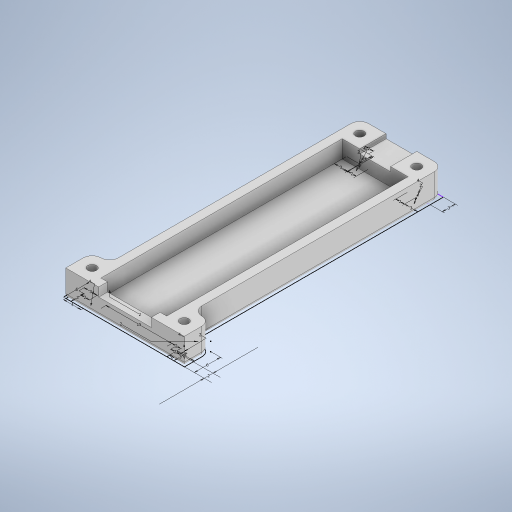
# Autodesk Inventor part: Case Atas
Saved by Autodesk Inventor 2024 (Build 280153000, 153)
## iProperties
Created: 2023-08-08
Part Number: Case Atas
Material: Generic
Document SubType Name: Modeling
Designer: Asus
Density: 1 g/cm^3
Appearance: Default
Author: Asus
## iProperties of the stored document Case Atas_3DPrint.ipt
Created: 2023-08-08
Part Number: Case Atas_3DPrint
Material: Generic
Document SubType Name: Modeling
Designer: Asus
Density: 1 g/cm^3
Appearance: Default
Author: Asus
Autodesk Inventor part; units mm, degrees
(part 1 of 2)
ref_plane "YZ Plane" through (0, 0, 0) normal (1, 0, 0) x (0, 1, 0)
ref_plane "XZ Plane" through (0, 0, 0) normal (0, 1, 0) x (-1, 0, 0)
ref_plane "XY Plane" through (0, 0, 0) normal (0, 0, 1) x (1, 0, 0)
sketch "Sketch2" plane through (0, 0, 0) normal (0, 1, 0) x (-1, 0, 0)
  line L0 (0, 0) -> (0, -2)
  line L1 (0, -2) -> (2, -2) construction
  line L2 (2, -2) -> (17, -2) construction
  line L3 (17, -2) -> (17, -57) construction
  line L4 (2, -2) -> (17, -2)
  line L5 (17, -2) -> (17, -57)
  line L6 (17, -57) -> (2, -57)
  line L7 (2, -57) -> (2, -2)
  line L8 (17, -57) -> (17, -63) construction
  line L9 (17, -63) -> (19, -63) construction
  line L10 (0, 0) -> (19, 0)
  line L11 (19, -8) -> (19, -63)
  line L12 (19, -63) -> (0, -63)
  line L13 (0, -63) -> (0, -8)
  line L14 (19, 0) -> (23, 0)
  line L15 (23, 0) -> (23, -4)
  line L16 (21, -6) -> (21, -6)
  arc A0 (21, -6) -> (19, -8) centre (21, -8) ccw
  arc A1 (21, -6) -> (23, -4) centre (21, -4) ccw
  line L17 (0, 0) -> (-4, 0)
  line L18 (-4, 0) -> (-4, -4)
  line L19 (-2, -6) -> (-2, -6)
  arc A2 (0, -8) -> (-2, -6) centre (-2, -8) ccw
  arc A3 (-4, -4) -> (-2, -6) centre (-2, -4) ccw
  line L20 (23, 0) -> (23, -3) construction
  line L21 (0, 0) -> (-1, 0) construction
  line L22 (-1, 0) -> (-1, -3) construction
  circle A4 centre (-1, -3) radius 1
  line L23 (23, 0) -> (23, -3) construction
  line L24 (23, -3) -> (20, -3) construction
  line L25 (20, -3) -> (22, -3) construction
  circle A5 centre (20, -3) radius 1
  line L26 (-1, -3) -> (1, -3) construction
  line L27 (0, -63) -> (0, -60) construction
  line L28 (0, -60) -> (3, -60) construction
  line L29 (19, -63) -> (19, -60) construction
  line L30 (19, -60) -> (16, -60) construction
  line L31 (16, -60) -> (14, -60) construction
  line L32 (3, -60) -> (5, -60) construction
  circle A6 centre (3, -60) radius 1
  circle A7 centre (16, -60) radius 1
  circle A8 centre (-1, -3) radius 2
  circle A9 centre (20, -3) radius 2
  circle A10 centre (3, -60) radius 2
  circle A11 centre (16, -60) radius 2
  point P0 (23, -6)
  point P1 (-4, -6)
  dimension "d4" = 2
  dimension "d5" = 2
  dimension "d6" = 15
  dimension "d8" = 6
  dimension "d9" = 2
  dimension "d15" = 4
  dimension "d16" = 6
  dimension "d17" = 2
  dimension "d18" = 4
  dimension "d19" = 6
  dimension "d20" = 2
  dimension "d34" = 1
  dimension "d35" = 3
  dimension "d36" = 2
  dimension "d39" = 3
  dimension "d40" = 3
  dimension "d41" = 2
  dimension "d43" = 2
  dimension "d52" = 3
  dimension "d53" = 3
  dimension "d54" = 3
  dimension "d55" = 3
  dimension "d56" = 2
  dimension "d57" = 2
  dimension "d58" = 2
  dimension "d59" = 2
  dimension "d73" = 4
  dimension "d74" = 4
  dimension "d75" = 4
  dimension "d76" = 4
  constraints: 66 end point, 15 point on line, 13 perpendicular, 12 centre point, 12 coincident, 8 point on circle, 8 tangent, 5 horizontal, 4 parallel, 2 equal radius, 2 vertical
  measures "d4" distance of L0.start L0.end
  measures "d5" distance of L0.end L1.end
  measures "d6" distance of L1.end L2.end
  measures "d8" distance of L3.end L8.end
  measures "d9" distance of L8.end L9.end
  measures "d15" distance of L10.end L14.end
  measures "d16" distance of L14.end point (23, -6)
  measures "d17" radius of A0
  measures "d18" distance of L0.start L17.end
  measures "d19" distance of L17.end point (-4, -6)
  measures "d20" radius of A2
  measures "d34" distance of L0.start L21.end
  measures "d35" distance of L21.end L22.end
  measures "d36" diameter of A4
  measures "d39" distance of L14.end L20.end
  measures "d40" distance of L20.end L24.end
  measures "d41" distance of L24.end L25.end
  measures "d43" distance of L26.start L26.end
  measures "d52" distance of L12.end L27.end
  measures "d53" distance of L27.end L28.end
  measures "d54" distance of L9.end L29.end
  measures "d55" distance of L29.end L30.end
  measures "d56" distance of L30.end L31.end
  measures "d57" distance of L28.end L32.end
  measures "d58" diameter of A6
  measures "d59" diameter of A7
  measures "d73" diameter of A8
  measures "d74" diameter of A9
  measures "d75" diameter of A10
  measures "d76" diameter of A11
extrude "Extrusion7" add sketch "Sketch2" along normal blind 6 contours L10 L14 L15 A1 A0 L11 L12 L13 A2 A3 L18 L17 | A4 | A5 | A8 | A9 | A10 | A11
extrude "Extrusion9" add sketch "Sketch2" along normal blind 2 contours L4 L5 L6 L7
sketch "Sketch7" plane through (-23, 0, 0) normal (0, 0, 1) x (1, 0, 0)
  line L0 (0, 0) -> (0, 6) construction
  line L1 (0, 6) -> (27, 6) construction
  line L2 (0, 6) -> (27, 6) construction
  line L3 (13.5, 6) -> (13.5, 4) construction
  line L4 (13.5, 4) -> (19.5, 4) construction
  line L5 (19.5, 4) -> (7.5, 4)
  line L6 (7.5, 4) -> (7.5, 6)
  line L7 (7.5, 6) -> (19.5, 6)
  line L8 (19.5, 6) -> (19.5, 4)
  point P0 (23, 0)
  dimension "d62" = 2
  dimension "d63" = 6
  dimension "d64" = 12
  constraints: 14 end point, 3 parallel, 1 collinear, 1 horizontal, 1 midpoint, 1 perpendicular, 1 point on line, 1 vertical
  measures "d62" distance of L3.start L3.end
  measures "d63" distance of L3.end L4.end
  measures "d64" distance of L6.end L7.end
extrude "Extrusion10" cut sketch "Sketch7" against normal blind 2
sketch "Sketch9" plane through (0, 0, -63) normal (0, 0, -1) x (-1, 0, 0)
  line L0 (0, 0) -> (0, 6) construction
  line L1 (0, 6) -> (19, 6) construction
  line L2 (0, 6) -> (19, 6) construction
  line L3 (9.5, 6) -> (9.5, 5) construction
  line L4 (9.5, 5) -> (13, 5) construction
  line L5 (13, 5) -> (6, 5)
  line L6 (6, 5) -> (6, 6)
  line L7 (6, 6) -> (13, 6)
  line L8 (13, 6) -> (13, 5)
  dimension "d67" = 1
  dimension "d68" = 3.5
  dimension "d69" = 7
  constraints: 14 end point, 3 equal length, 2 perpendicular, 1 horizontal, 1 midpoint, 1 point on line, 1 vertical
  measures "d67" distance of L3.start L3.end
  measures "d68" distance of L3.end L4.end
  measures "d69" distance of L6.end L7.end
extrude "Extrusion11" cut sketch "Sketch9" against normal blind 6
fillet "Fillet1" radius 2 2 edges at (0, 3, -63) (-19, 3, -63)
extrude "Extrusion12" cut sketch "Sketch2" along normal blind 1 contours A4 | A5 | A6 | A7 | A8 | A9 | A10 | A11
extrude "Extrusion13" cut sketch "Sketch2" along normal blind 6 contours A4 | A5
fillet "Fillet2" radius 0.9 12 edges at (-0.5858, 0, -62.4142) (-9.5, 0, -63) (-18.4142, 0, -62.4142) (-19, 0, -34.5) (-19.5858, 0, -6.5858) (-22.4142, 0, -5.4142) (-23, 0, -2) (0.5858, 0, -6.5858) (3.4142, 0, -5.4142) (4, 0, -2) (0, 0, -34.5) (-9.5, 0, 0)
sketch "Sketch10" plane through (0, 0, 0) normal (0, -1, 0) x (1, 0, 0)
  line L0 (-5.0264, -9.1176) -> (-5.0264, -52.1576) construction
  line L1 (-5.0264, -52.1576) -> (-18.2298, -52.1576) construction
  line L2 (-18.2298, -52.1576) -> (-18.2298, -9.1176) construction
  line L3 (-18.2298, -9.1176) -> (-5.0264, -9.1176) construction
  line L4 (-5.0599, -17.9524) -> (-5.0599, -18.3563)
  line L5 (-5.0599, -18.3563) -> (-6.1437, -18.3563)
  spline S0 degree 2 poles (-6.1437, -18.3563) (-6.4014, -18.3563) (-6.4776, -18.3716) knots 0 0 0 1 1 1
  spline S1 degree 2 poles (-6.4776, -18.3716) (-6.5995, -18.3975) (-6.7489, -18.5926) (-6.7489, -18.7618) knots 0 0 0 1 2 2 2
  spline S2 degree 2 poles (-6.7489, -18.7618) (-6.7489, -18.9326) (-6.6087, -19.1079) (-6.4044, -19.1429) (-6.1666, -19.1429) knots 0 0 0 1 2 3 3 3
  line L6 (-6.1666, -19.1429) -> (-5.0599, -19.1429)
  line L7 (-5.0599, -19.1429) -> (-5.0599, -19.5469)
  line L8 (-5.0599, -19.5469) -> (-6.1102, -19.5469)
  spline S3 degree 2 poles (-6.1102, -19.5469) (-6.47, -19.5469) (-6.7672, -19.4813) (-6.9715, -19.306) (-7.0934, -19.0103) (-7.0934, -18.774) knots 0 0 0 1 2 3 4 4 4
  spline S4 degree 2 poles (-7.0934, -18.774) (-7.0934, -18.4874) (-6.9608, -18.1917) (-6.7504, -18.0194) (-6.6331, -17.992) knots 0 0 0 1 2 3 3 3
  spline S5 degree 2 poles (-6.6331, -17.992) (-6.4623, -17.9524) (-6.127, -17.9524) knots 0 0 0 1 1 1
  line L9 (-6.127, -17.9524) -> (-5.0599, -17.9524)
  line L10 (-6.4075, -19.8701) -> (-6.3693, -20.2633)
  spline S6 degree 2 poles (-6.3693, -20.2633) (-6.5675, -20.2984) (-6.7535, -20.5164) (-6.7535, -20.6993) knots 0 0 0 1 2 2 2
  spline S7 degree 2 poles (-6.7535, -20.6993) (-6.7535, -20.8944) (-6.5889, -21.0926) (-6.4776, -21.0926) knots 0 0 0 1 2 2 2
  spline S8 degree 2 poles (-6.4776, -21.0926) (-6.4059, -21.0926) (-6.3068, -21.0088) (-6.2703, -20.9051) knots 0 0 0 1 2 2 2
  spline S9 degree 2 poles (-6.2703, -20.9051) (-6.2459, -20.835) (-6.1834, -20.5819) knots 0 0 0 1 1 1
  spline S10 degree 2 poles (-6.1834, -20.5819) (-6.1026, -20.2572) (-5.9852, -20.1262) knots 0 0 0 1 1 1
  spline S11 degree 2 poles (-5.9852, -20.1262) (-5.8206, -19.9417) (-5.5843, -19.9417) knots 0 0 0 1 1 1
  spline S12 degree 2 poles (-5.5843, -19.9417) (-5.4303, -19.9417) (-5.1651, -20.1155) (-5.0264, -20.4417) (-5.0264, -20.6719) knots 0 0 0 1 2 3 3 3
  spline S13 degree 2 poles (-5.0264, -20.6719) (-5.0264, -21.0484) (-5.3556, -21.4295) (-5.6315, -21.4387) knots 0 0 0 1 2 2 2
  line L11 (-5.6315, -21.4387) -> (-5.6498, -21.0347)
  spline S14 degree 2 poles (-5.6498, -21.0347) (-5.4959, -21.0088) (-5.3602, -20.838) (-5.3602, -20.6673) knots 0 0 0 1 2 2 2
  spline S15 degree 2 poles (-5.3602, -20.6673) (-5.3602, -20.4905) (-5.4318, -20.3914) knots 0 0 0 1 1 1
  spline S16 degree 2 poles (-5.4318, -20.3914) (-5.4791, -20.3274) (-5.5568, -20.3274) knots 0 0 0 1 1 1
  spline S17 degree 2 poles (-5.5568, -20.3274) (-5.627, -20.3274) (-5.6788, -20.3868) knots 0 0 0 1 1 1
  spline S18 degree 2 poles (-5.6788, -20.3868) (-5.7428, -20.4646) (-5.8815, -21.0545) (-6.0294, -21.3365) (-6.287, -21.4966) (-6.4776, -21.4966) knots 0 0 0 1 2 3 4 4 4
  spline S19 degree 2 poles (-6.4776, -21.4966) (-6.6483, -21.4966) (-6.9486, -21.306) (-7.095, -20.9569) (-7.095, -20.6963) knots 0 0 0 1 2 3 3 3
  spline S20 degree 2 poles (-7.095, -20.6963) (-7.095, -20.3167) (-6.7443, -19.9097) (-6.4075, -19.8701) knots 0 0 0 1 2 2 2
  line L12 (-5.0599, -21.838) -> (-5.0599, -22.6383)
  spline S21 degree 2 poles (-5.0599, -22.6383) (-5.0599, -22.8762) (-5.0995, -23.1094) (-5.2245, -23.2938) (-5.4334, -23.4173) (-5.5629, -23.4173) knots 0 0 0 1 2 3 4 4 4
  spline S22 degree 2 poles (-5.5629, -23.4173) (-5.7032, -23.4173) (-5.9364, -23.2664) (-5.9959, -23.1368) knots 0 0 0 1 2 2 2
  spline S23 degree 2 poles (-5.9959, -23.1368) (-6.0492, -23.3197) (-6.3053, -23.5149) (-6.4791, -23.5149) knots 0 0 0 1 2 2 2
  spline S24 degree 2 poles (-6.4791, -23.5149) (-6.6163, -23.5149) (-6.8739, -23.3883) (-7.0279, -23.1673) (-7.0462, -23.0072) knots 0 0 0 1 2 3 3 3
  spline S25 degree 2 poles (-7.0462, -23.0072) (-7.0568, -22.9051) (-7.0599, -22.5194) knots 0 0 0 1 1 1
  line L13 (-7.0599, -22.5194) -> (-7.0599, -21.838)
  line L14 (-7.0599, -21.838) -> (-5.0599, -21.838)
  line L15 (-6.1864, -22.242) -> (-6.7215, -22.242)
  line L16 (-6.7215, -22.242) -> (-6.7215, -22.617)
  spline S26 degree 2 poles (-6.7215, -22.617) (-6.7215, -22.8365) (-6.7093, -22.8944) knots 0 0 0 1 1 1
  spline S27 degree 2 poles (-6.7093, -22.8944) (-6.6925, -22.9844) (-6.566, -23.0987) (-6.4593, -23.0987) knots 0 0 0 1 2 2 2
  spline S28 degree 2 poles (-6.4593, -23.0987) (-6.3693, -23.0987) (-6.2443, -23.0118) (-6.1864, -22.8457) (-6.1864, -22.5697) knots 0 0 0 1 2 3 3 3
  line L17 (-6.1864, -22.5697) -> (-6.1864, -22.242)
  line L18 (-5.3922, -22.242) -> (-5.8541, -22.242)
  line L19 (-5.8541, -22.242) -> (-5.8541, -22.5072)
  spline S29 degree 2 poles (-5.8541, -22.5072) (-5.8541, -22.7435) (-5.848, -22.8015) knots 0 0 0 1 1 1
  spline S30 degree 2 poles (-5.848, -22.8015) (-5.8343, -22.9051) (-5.7169, -23.024) (-5.6193, -23.024) knots 0 0 0 1 2 2 2
  spline S31 degree 2 poles (-5.6193, -23.024) (-5.5264, -23.024) (-5.412, -22.9219) (-5.3983, -22.8197) knots 0 0 0 1 2 2 2
  spline S32 degree 2 poles (-5.3983, -22.8197) (-5.3922, -22.7603) (-5.3922, -22.4737) knots 0 0 0 1 1 1
  line L20 (-5.3922, -22.4737) -> (-5.3922, -22.242)
  line L21 (-5.6102, -25.2923) -> (-5.9151, -25.2923)
  line L22 (-5.9151, -25.2923) -> (-5.9151, -25.0301)
  line L23 (-5.9151, -25.0301) -> (-6.4989, -25.0301)
  spline S33 degree 2 poles (-6.4989, -25.0301) (-6.6757, -25.0301) (-6.7352, -25.0454) (-6.7733, -25.0987) (-6.7733, -25.1368) knots 0 0 0 1 2 3 3 3
  spline S34 degree 2 poles (-6.7733, -25.1368) (-6.7733, -25.1902) (-6.7367, -25.2923) knots 0 0 0 1 1 1
  line L24 (-6.7367, -25.2923) -> (-7.034, -25.3243)
  spline S35 degree 2 poles (-7.034, -25.3243) (-7.0919, -25.1902) (-7.0919, -25.021) knots 0 0 0 1 1 1
  spline S36 degree 2 poles (-7.0919, -25.021) (-7.0919, -24.9173) (-7.0218, -24.7512) (-6.912, -24.6734) (-6.8175, -24.6582) knots 0 0 0 1 2 3 3 3
  spline S37 degree 2 poles (-6.8175, -24.6582) (-6.7504, -24.646) (-6.5477, -24.646) knots 0 0 0 1 1 1
  line L25 (-6.5477, -24.646) -> (-5.9151, -24.646)
  line L26 (-5.9151, -24.646) -> (-5.9151, -24.4707)
  line L27 (-5.9151, -24.4707) -> (-5.6102, -24.4707)
  line L28 (-5.6102, -24.4707) -> (-5.6102, -24.646)
  line L29 (-5.6102, -24.646) -> (-5.3221, -24.646)
  line L30 (-5.3221, -24.646) -> (-5.0965, -25.0301)
  line L31 (-5.0965, -25.0301) -> (-5.6102, -25.0301)
  line L32 (-5.6102, -25.0301) -> (-5.6102, -25.2923)
  spline S38 degree 2 poles (-6.3145, -25.4691) (-6.1239, -25.4691) (-5.7657, -25.6582) (-5.5782, -26.0027) (-5.5782, -26.2161) knots 0 0 0 1 2 3 3 3
  spline S39 degree 2 poles (-5.5782, -26.2161) (-5.5782, -26.5454) (-6.005, -26.9661) (-6.3312, -26.9661) knots 0 0 0 1 2 2 2
  spline S40 degree 2 poles (-6.3312, -26.9661) (-6.659, -26.9661) (-7.0919, -26.5408) (-7.0919, -26.2191) knots 0 0 0 1 2 2 2
  spline S41 degree 2 poles (-7.0919, -26.2191) (-7.0919, -26.0194) (-6.912, -25.6582) (-6.5645, -25.4691) (-6.3145, -25.4691) knots 0 0 0 1 2 3 3 3
  spline S42 degree 2 poles (-6.3343, -25.8624) (-6.5507, -25.8624) (-6.7794, -26.0667) (-6.7794, -26.2176) knots 0 0 0 1 2 2 2
  spline S43 degree 2 poles (-6.7794, -26.2176) (-6.7794, -26.3685) (-6.5507, -26.5713) (-6.3328, -26.5713) knots 0 0 0 1 2 2 2
  spline S44 degree 2 poles (-6.3328, -26.5713) (-6.1193, -26.5713) (-5.8907, -26.3685) (-5.8907, -26.2176) knots 0 0 0 1 2 2 2
  spline S45 degree 2 poles (-5.8907, -26.2176) (-5.8907, -26.0667) (-6.1193, -25.8624) (-6.3343, -25.8624) knots 0 0 0 1 2 2 2
  line L33 (-7.0599, -28.4951) -> (-5.3983, -28.4951)
  line L34 (-5.3983, -28.4951) -> (-5.3983, -27.9021)
  line L35 (-5.3983, -27.9021) -> (-5.0599, -27.9021)
  line L36 (-5.0599, -27.9021) -> (-5.0599, -29.4905)
  line L37 (-5.0599, -29.4905) -> (-5.3983, -29.4905)
  line L38 (-5.3983, -29.4905) -> (-5.3983, -28.899)
  line L39 (-5.3983, -28.899) -> (-7.0599, -28.899)
  line L40 (-7.0599, -28.899) -> (-7.0599, -28.4951)
  line L41 (-7.0599, -30.2024) -> (-5.3983, -30.2024)
  line L42 (-5.3983, -30.2024) -> (-5.3983, -29.6094)
  line L43 (-5.3983, -29.6094) -> (-5.0599, -29.6094)
  line L44 (-5.0599, -29.6094) -> (-5.0599, -31.1978)
  line L45 (-5.0599, -31.1978) -> (-5.3983, -31.1978)
  line L46 (-5.3983, -31.1978) -> (-5.3983, -30.6063)
  line L47 (-5.3983, -30.6063) -> (-7.0599, -30.6063)
  line L48 (-7.0599, -30.6063) -> (-7.0599, -30.2024)
  line L49 (-7.0599, -31.4707) -> (-5.0767, -31.4707)
  line L50 (-5.0767, -31.4707) -> (-5.0767, -31.8746)
  line L51 (-5.0767, -31.8746) -> (-6.7215, -31.8746)
  line L52 (-6.7215, -31.8746) -> (-6.7215, -32.8792)
  line L53 (-6.7215, -32.8792) -> (-7.0599, -32.8792)
  line L54 (-7.0599, -32.8792) -> (-7.0599, -31.4707)
  line L55 (-7.0599, -33.9432) -> (-5.0599, -33.9432)
  line L56 (-5.0599, -33.9432) -> (-5.0599, -34.5911)
  spline S46 degree 2 poles (-5.0599, -34.5911) (-5.0599, -34.96) (-5.0904, -35.0713) knots 0 0 0 1 1 1
  spline S47 degree 2 poles (-5.0904, -35.0713) (-5.1346, -35.2435) (-5.4364, -35.4752) (-5.6757, -35.4752) knots 0 0 0 1 2 2 2
  spline S48 degree 2 poles (-5.6757, -35.4752) (-5.8587, -35.4752) (-6.1102, -35.3411) (-6.2535, -35.1353) (-6.2764, -35.0286) knots 0 0 0 1 2 3 3 3
  spline S49 degree 2 poles (-6.2764, -35.0286) (-6.3053, -34.8853) (-6.3053, -34.6109) knots 0 0 0 1 1 1
  line L57 (-6.3053, -34.6109) -> (-6.3053, -34.3472)
  line L58 (-6.3053, -34.3472) -> (-7.0599, -34.3472)
  line L59 (-7.0599, -34.3472) -> (-7.0599, -33.9432)
  line L60 (-5.3983, -34.3472) -> (-5.9669, -34.3472)
  line L61 (-5.9669, -34.3472) -> (-5.9669, -34.5682)
  spline S50 degree 2 poles (-5.9669, -34.5682) (-5.9669, -34.8076) (-5.9044, -34.9676) (-5.7703, -35.0591) (-5.6818, -35.0591) knots 0 0 0 1 2 3 3 3
  spline S51 degree 2 poles (-5.6818, -35.0591) (-5.5721, -35.0591) (-5.4303, -34.931) (-5.412, -34.8319) knots 0 0 0 1 2 2 2
  spline S52 degree 2 poles (-5.412, -34.8319) (-5.3983, -34.7603) (-5.3983, -34.5423) knots 0 0 0 1 1 1
  line L62 (-5.3983, -34.5423) -> (-5.3983, -34.3472)
  line L63 (-7.0599, -35.8182) -> (-5.0767, -35.8182)
  line L64 (-5.0767, -35.8182) -> (-5.0767, -36.2222)
  line L65 (-5.0767, -36.2222) -> (-6.7215, -36.2222)
  line L66 (-6.7215, -36.2222) -> (-6.7215, -37.2268)
  line L67 (-6.7215, -37.2268) -> (-7.0599, -37.2268)
  line L68 (-7.0599, -37.2268) -> (-7.0599, -35.8182)
  line L69 (-6.7032, -38.7237) -> (-7.0599, -38.7237)
  line L70 (-7.0599, -38.7237) -> (-7.0599, -37.3807)
  spline S53 degree 2 poles (-7.0599, -37.3807) (-6.8587, -37.4021) (-6.4974, -37.6201) (-6.1986, -37.9432) knots 0 0 0 1 2 2 2
  spline S54 degree 2 poles (-6.1986, -37.9432) (-5.9578, -38.2024) (-5.8709, -38.2603) knots 0 0 0 1 1 1
  spline S55 degree 2 poles (-5.8709, -38.2603) (-5.752, -38.3396) (-5.6361, -38.3396) knots 0 0 0 1 1 1
  spline S56 degree 2 poles (-5.6361, -38.3396) (-5.5081, -38.3396) (-5.3709, -38.2024) (-5.3709, -38.0804) knots 0 0 0 1 2 2 2
  spline S57 degree 2 poles (-5.3709, -38.0804) (-5.3709, -37.9615) (-5.5157, -37.8197) (-5.6834, -37.8091) knots 0 0 0 1 2 2 2
  line L71 (-5.6834, -37.8091) -> (-5.6453, -37.4265)
  spline S58 degree 2 poles (-5.6453, -37.4265) (-5.3282, -37.46) (-5.0523, -37.8197) (-5.0523, -38.0896) knots 0 0 0 1 2 2 2
  spline S59 degree 2 poles (-5.0523, -38.0896) (-5.0523, -38.3853) (-5.3709, -38.7237) (-5.6087, -38.7237) knots 0 0 0 1 2 2 2
  spline S60 degree 2 poles (-5.6087, -38.7237) (-5.7428, -38.7237) (-5.9867, -38.6277) (-6.1209, -38.5225) knots 0 0 0 1 2 2 2
  spline S61 degree 2 poles (-6.1209, -38.5225) (-6.2093, -38.4524) (-6.5416, -38.0896) (-6.6514, -37.992) (-6.7032, -37.963) knots 0 0 0 1 2 3 3 3
  line L72 (-6.7032, -37.963) -> (-6.7032, -38.7237)
  line L73 (-6.5279, -38.9691) -> (-6.4821, -39.3396)
  spline S62 degree 2 poles (-6.4821, -39.3396) (-6.6239, -39.3579) (-6.7748, -39.5133) (-6.7748, -39.6231) knots 0 0 0 1 2 2 2
  spline S63 degree 2 poles (-6.7748, -39.6231) (-6.7748, -39.742) (-6.595, -39.9036) (-6.4425, -39.9036) knots 0 0 0 1 2 2 2
  spline S64 degree 2 poles (-6.4425, -39.9036) (-6.2977, -39.9036) (-6.1285, -39.7496) (-6.1285, -39.6383) knots 0 0 0 1 2 2 2
  spline S65 degree 2 poles (-6.1285, -39.6383) (-6.1285, -39.5652) (-6.1575, -39.463) knots 0 0 0 1 1 1
  line L74 (-6.1575, -39.463) -> (-5.845, -39.5057)
  spline S66 degree 2 poles (-5.845, -39.5057) (-5.8495, -39.6612) (-5.7062, -39.8243) (-5.5873, -39.8243) knots 0 0 0 1 2 2 2
  spline S67 degree 2 poles (-5.5873, -39.8243) (-5.4867, -39.8243) (-5.3678, -39.7039) (-5.3678, -39.6048) knots 0 0 0 1 2 2 2
  spline S68 degree 2 poles (-5.3678, -39.6048) (-5.3678, -39.5057) (-5.5035, -39.367) (-5.6346, -39.3518) knots 0 0 0 1 2 2 2
  line L75 (-5.6346, -39.3518) -> (-5.5751, -38.9981)
  spline S69 degree 2 poles (-5.5751, -38.9981) (-5.3937, -39.0347) (-5.1757, -39.1841) (-5.0523, -39.4493) (-5.0523, -39.6155) knots 0 0 0 1 2 3 3 3
  spline S70 degree 2 poles (-5.0523, -39.6155) (-5.0523, -39.8975) (-5.2321, -40.0682) knots 0 0 0 1 1 1
  spline S71 degree 2 poles (-5.2321, -40.0682) (-5.3785, -40.2085) (-5.5645, -40.2085) knots 0 0 0 1 1 1
  spline S72 degree 2 poles (-5.5645, -40.2085) (-5.8267, -40.2085) (-5.9837, -39.9204) knots 0 0 0 1 1 1
  spline S73 degree 2 poles (-5.9837, -39.9204) (-6.0203, -40.0926) (-6.2779, -40.2969) (-6.4593, -40.2969) knots 0 0 0 1 2 2 2
  spline S74 degree 2 poles (-6.4593, -40.2969) (-6.723, -40.2969) (-7.0934, -39.9127) (-7.0934, -39.6262) knots 0 0 0 1 2 2 2
  spline S75 degree 2 poles (-7.0934, -39.6262) (-7.0934, -39.3548) (-6.7809, -38.9981) (-6.5279, -38.9691) knots 0 0 0 1 2 2 2
  spline S76 degree 2 poles (-5.0523, -41.1841) (-5.0523, -41.4752) (-5.2596, -41.6383) knots 0 0 0 1 1 1
  spline S77 degree 2 poles (-5.2596, -41.6383) (-5.505, -41.8335) (-6.0736, -41.8335) knots 0 0 0 1 1 1
  spline S78 degree 2 poles (-6.0736, -41.8335) (-6.6407, -41.8335) (-6.8892, -41.6368) knots 0 0 0 1 1 1
  spline S79 degree 2 poles (-6.8892, -41.6368) (-7.0934, -41.4752) (-7.0934, -41.1841) knots 0 0 0 1 1 1
  spline S80 degree 2 poles (-7.0934, -41.1841) (-7.0934, -40.8914) (-6.6453, -40.5347) (-6.069, -40.5347) knots 0 0 0 1 2 2 2
  spline S81 degree 2 poles (-6.069, -40.5347) (-5.505, -40.5347) (-5.2565, -40.7313) knots 0 0 0 1 1 1
  spline S82 degree 2 poles (-5.2565, -40.7313) (-5.0523, -40.8929) (-5.0523, -41.1841) knots 0 0 0 1 1 1
  spline S83 degree 2 poles (-5.3709, -41.1841) (-5.3709, -41.114) (-5.4593, -41.0057) (-5.5736, -40.9752) knots 0 0 0 1 2 2 2
  spline S84 degree 2 poles (-5.5736, -40.9752) (-5.7215, -40.9356) (-6.0736, -40.9356) knots 0 0 0 1 1 1
  spline S85 degree 2 poles (-6.0736, -40.9356) (-6.4242, -40.9356) (-6.6879, -41.0072) (-6.7748, -41.114) (-6.7748, -41.1841) knots 0 0 0 1 2 3 3 3
  spline S86 degree 2 poles (-6.7748, -41.1841) (-6.7748, -41.2542) (-6.6864, -41.3624) (-6.5721, -41.3929) knots 0 0 0 1 2 2 2
  spline S87 degree 2 poles (-6.5721, -41.3929) (-6.4242, -41.4326) (-6.0736, -41.4326) knots 0 0 0 1 1 1
  spline S88 degree 2 poles (-6.0736, -41.4326) (-5.7215, -41.4326) (-5.4593, -41.3609) (-5.3709, -41.2542) (-5.3709, -41.1841) knots 0 0 0 1 2 3 3 3
  line L76 (-6.5279, -42.0758) -> (-6.4821, -42.4463)
  spline S89 degree 2 poles (-6.4821, -42.4463) (-6.6239, -42.4646) (-6.7748, -42.6201) (-6.7748, -42.7298) knots 0 0 0 1 2 2 2
  spline S90 degree 2 poles (-6.7748, -42.7298) (-6.7748, -42.8487) (-6.595, -43.0103) (-6.4425, -43.0103) knots 0 0 0 1 2 2 2
  spline S91 degree 2 poles (-6.4425, -43.0103) (-6.2977, -43.0103) (-6.1285, -42.8563) (-6.1285, -42.7451) knots 0 0 0 1 2 2 2
  spline S92 degree 2 poles (-6.1285, -42.7451) (-6.1285, -42.6719) (-6.1575, -42.5697) knots 0 0 0 1 1 1
  line L77 (-6.1575, -42.5697) -> (-5.845, -42.6124)
  spline S93 degree 2 poles (-5.845, -42.6124) (-5.8495, -42.7679) (-5.7062, -42.931) (-5.5873, -42.931) knots 0 0 0 1 2 2 2
  spline S94 degree 2 poles (-5.5873, -42.931) (-5.4867, -42.931) (-5.3678, -42.8106) (-5.3678, -42.7115) knots 0 0 0 1 2 2 2
  spline S95 degree 2 poles (-5.3678, -42.7115) (-5.3678, -42.6124) (-5.5035, -42.4737) (-5.6346, -42.4585) knots 0 0 0 1 2 2 2
  line L78 (-5.6346, -42.4585) -> (-5.5751, -42.1048)
  spline S96 degree 2 poles (-5.5751, -42.1048) (-5.3937, -42.1414) (-5.1757, -42.2908) (-5.0523, -42.556) (-5.0523, -42.7222) knots 0 0 0 1 2 3 3 3
  spline S97 degree 2 poles (-5.0523, -42.7222) (-5.0523, -43.0042) (-5.2321, -43.1749) knots 0 0 0 1 1 1
  spline S98 degree 2 poles (-5.2321, -43.1749) (-5.3785, -43.3152) (-5.5645, -43.3152) knots 0 0 0 1 1 1
  spline S99 degree 2 poles (-5.5645, -43.3152) (-5.8267, -43.3152) (-5.9837, -43.0271) knots 0 0 0 1 1 1
  spline S100 degree 2 poles (-5.9837, -43.0271) (-6.0203, -43.1993) (-6.2779, -43.4036) (-6.4593, -43.4036) knots 0 0 0 1 2 2 2
  spline S101 degree 2 poles (-6.4593, -43.4036) (-6.723, -43.4036) (-7.0934, -43.0194) (-7.0934, -42.7329) knots 0 0 0 1 2 2 2
  spline S102 degree 2 poles (-7.0934, -42.7329) (-7.0934, -42.4615) (-6.7809, -42.1048) (-6.5279, -42.0758) knots 0 0 0 1 2 2 2
  line L79 (-10.2073, -15.2519) -> (-8.2241, -15.2519)
  line L80 (-8.2241, -15.2519) -> (-8.2241, -15.6559)
  line L81 (-8.2241, -15.6559) -> (-9.8689, -15.6559)
  line L82 (-9.8689, -15.6559) -> (-9.8689, -16.6604)
  line L83 (-9.8689, -16.6604) -> (-10.2073, -16.6604)
  line L84 (-10.2073, -16.6604) -> (-10.2073, -15.2519)
  line L85 (-9.1997, -17.2306) -> (-9.1372, -16.883)
  spline S103 degree 2 poles (-9.1372, -16.883) (-8.9268, -16.9425) (-8.7256, -17.229) (-8.7256, -17.5111) knots 0 0 0 1 2 2 2
  spline S104 degree 2 poles (-8.7256, -17.5111) (-8.7256, -17.7687) (-8.8475, -18.0202) (-9.0335, -18.1223) (-9.2835, -18.1223) knots 0 0 0 1 2 3 3 3
  line L86 (-9.2835, -18.1223) -> (-9.7317, -18.1162)
  spline S105 degree 2 poles (-9.7317, -18.1162) (-9.9222, -18.1162) (-10.1036, -18.1528) (-10.2073, -18.2031) knots 0 0 0 1 2 2 2
  line L87 (-10.2073, -18.2031) -> (-10.2073, -17.8236)
  spline S106 degree 2 poles (-10.2073, -17.8236) (-10.1692, -17.8083) (-10.0945, -17.787) knots 0 0 0 1 1 1
  spline S107 degree 2 poles (-10.0945, -17.787) (-10.0594, -17.7778) (-10.0488, -17.7733) knots 0 0 0 1 1 1
  spline S108 degree 2 poles (-10.0488, -17.7733) (-10.1433, -17.6757) (-10.2393, -17.4516) (-10.2393, -17.3251) knots 0 0 0 1 2 2 2
  spline S109 degree 2 poles (-10.2393, -17.3251) (-10.2393, -17.101) (-9.9969, -16.8434) (-9.811, -16.8434) knots 0 0 0 1 2 2 2
  spline S110 degree 2 poles (-9.811, -16.8434) (-9.6875, -16.8434) (-9.4954, -16.9608) (-9.3933, -17.1726) (-9.3552, -17.3723) knots 0 0 0 1 2 3 3 3
  spline S111 degree 2 poles (-9.3552, -17.3723) (-9.3049, -17.6406) (-9.2606, -17.7443) knots 0 0 0 1 1 1
  line L88 (-9.2606, -17.7443) -> (-9.2225, -17.7443)
  spline S112 degree 2 poles (-9.2225, -17.7443) (-9.1128, -17.7443) (-9.0183, -17.6345) (-9.0183, -17.4836) knots 0 0 0 1 2 2 2
  spline S113 degree 2 poles (-9.0183, -17.4836) (-9.0183, -17.3815) (-9.0991, -17.2656) (-9.1997, -17.2306) knots 0 0 0 1 2 2 2
  spline S114 degree 2 poles (-9.5106, -17.7443) (-9.535, -17.6711) (-9.6036, -17.351) (-9.6356, -17.3022) knots 0 0 0 1 2 2 2
  spline S115 degree 2 poles (-9.6356, -17.3022) (-9.689, -17.2275) (-9.7713, -17.2275) knots 0 0 0 1 1 1
  spline S116 degree 2 poles (-9.7713, -17.2275) (-9.8521, -17.2275) (-9.9695, -17.3479) (-9.9695, -17.4409) knots 0 0 0 1 2 2 2
  spline S117 degree 2 poles (-9.9695, -17.4409) (-9.9695, -17.5446) (-9.9009, -17.6376) knots 0 0 0 1 1 1
  spline S118 degree 2 poles (-9.9009, -17.6376) (-9.8491, -17.7077) (-9.7744, -17.729) knots 0 0 0 1 1 1
  spline S119 degree 2 poles (-9.7744, -17.729) (-9.7256, -17.7443) (-9.5869, -17.7443) knots 0 0 0 1 1 1
  line L89 (-9.5869, -17.7443) -> (-9.5106, -17.7443)
  line L90 (-10.2073, -18.4821) -> (-8.2073, -18.4821)
  line L91 (-8.2073, -18.4821) -> (-8.2073, -18.8662)
  line L92 (-8.2073, -18.8662) -> (-8.9268, -18.8662)
  spline S120 degree 2 poles (-8.9268, -18.8662) (-8.7256, -19.0431) (-8.7256, -19.2854) knots 0 0 0 1 1 1
  spline S121 degree 2 poles (-8.7256, -19.2854) (-8.7256, -19.5507) (-9.1082, -19.8967) (-9.468, -19.8967) knots 0 0 0 1 2 2 2
  spline S122 degree 2 poles (-9.468, -19.8967) (-9.8384, -19.8967) (-10.2393, -19.5431) (-10.2393, -19.2915) knots 0 0 0 1 2 2 2
  spline S123 degree 2 poles (-10.2393, -19.2915) (-10.2393, -19.1681) (-10.1158, -18.9257) (-9.9939, -18.8388) knots 0 0 0 1 2 2 2
  line L93 (-9.9939, -18.8388) -> (-10.2073, -18.8388)
  line L94 (-10.2073, -18.8388) -> (-10.2073, -18.4821)
  spline S124 degree 2 poles (-9.4512, -18.8632) (-9.6753, -18.8632) (-9.7835, -18.9333) knots 0 0 0 1 1 1
  spline S125 degree 2 poles (-9.7835, -18.9333) (-9.936, -19.0339) (-9.936, -19.1986) knots 0 0 0 1 1 1
  spline S126 degree 2 poles (-9.936, -19.1986) (-9.936, -19.3251) (-9.7195, -19.5034) (-9.4863, -19.5034) knots 0 0 0 1 2 2 2
  spline S127 degree 2 poles (-9.4863, -19.5034) (-9.2378, -19.5034) (-9.0183, -19.3236) (-9.0183, -19.1833) knots 0 0 0 1 2 2 2
  spline S128 degree 2 poles (-9.0183, -19.1833) (-9.0183, -19.0461) (-9.2317, -18.8632) (-9.4512, -18.8632) knots 0 0 0 1 2 2 2
  line L95 (-10.2073, -20.2047) -> (-9.8231, -20.2047)
  line L96 (-9.8231, -20.2047) -> (-9.8231, -20.5888)
  line L97 (-9.8231, -20.5888) -> (-10.2073, -20.5888)
  line L98 (-10.2073, -20.5888) -> (-10.2073, -20.2047)
  line L99 (-10.2073, -21.7656) -> (-8.2073, -21.7656)
  line L100 (-8.2073, -21.7656) -> (-8.2073, -22.1696)
  line L101 (-8.2073, -22.1696) -> (-9.096, -22.1696)
  line L102 (-9.096, -22.1696) -> (-8.2073, -22.9851)
  line L103 (-8.2073, -22.9851) -> (-8.2073, -23.5294)
  line L104 (-8.2073, -23.5294) -> (-8.9863, -22.7748)
  line L105 (-8.9863, -22.7748) -> (-10.2073, -23.5705)
  line L106 (-10.2073, -23.5705) -> (-10.2073, -23.0476)
  line L107 (-10.2073, -23.0476) -> (-9.2683, -22.4958)
  line L108 (-9.2683, -22.4958) -> (-9.6036, -22.1696)
  line L109 (-9.6036, -22.1696) -> (-10.2073, -22.1696)
  line L110 (-10.2073, -22.1696) -> (-10.2073, -21.7656)
  spline S129 degree 2 poles (-9.4619, -23.6864) (-9.2713, -23.6864) (-8.9131, -23.8754) (-8.7256, -24.2199) (-8.7256, -24.4333) knots 0 0 0 1 2 3 3 3
  spline S130 degree 2 poles (-8.7256, -24.4333) (-8.7256, -24.7626) (-9.1524, -25.1833) (-9.4786, -25.1833) knots 0 0 0 1 2 2 2
  spline S131 degree 2 poles (-9.4786, -25.1833) (-9.8064, -25.1833) (-10.2393, -24.758) (-10.2393, -24.4364) knots 0 0 0 1 2 2 2
  spline S132 degree 2 poles (-10.2393, -24.4364) (-10.2393, -24.2367) (-10.0594, -23.8754) (-9.7119, -23.6864) (-9.4619, -23.6864) knots 0 0 0 1 2 3 3 3
  spline S133 degree 2 poles (-9.4817, -24.0797) (-9.6981, -24.0797) (-9.9268, -24.2839) (-9.9268, -24.4348) knots 0 0 0 1 2 2 2
  spline S134 degree 2 poles (-9.9268, -24.4348) (-9.9268, -24.5858) (-9.6981, -24.7885) (-9.4802, -24.7885) knots 0 0 0 1 2 2 2
  spline S135 degree 2 poles (-9.4802, -24.7885) (-9.2667, -24.7885) (-9.0381, -24.5858) (-9.0381, -24.4348) knots 0 0 0 1 2 2 2
  spline S136 degree 2 poles (-9.0381, -24.4348) (-9.0381, -24.2839) (-9.2667, -24.0797) (-9.4817, -24.0797) knots 0 0 0 1 2 2 2
  line L111 (-10.2073, -26.8007) -> (-10.2073, -26.4165)
  line L112 (-10.2073, -26.4165) -> (-9.468, -26.4165)
  spline S137 degree 2 poles (-9.468, -26.4165) (-9.2332, -26.4165) (-9.0945, -26.3678) (-9.0183, -26.2565) (-9.0183, -26.1787) knots 0 0 0 1 2 3 3 3
  spline S138 degree 2 poles (-9.0183, -26.1787) (-9.0183, -26.0797) (-9.128, -25.9211) (-9.3079, -25.8632) (-9.5503, -25.8632) knots 0 0 0 1 2 3 3 3
  line L113 (-9.5503, -25.8632) -> (-10.2073, -25.8632)
  line L114 (-10.2073, -25.8632) -> (-10.2073, -25.479)
  line L115 (-10.2073, -25.479) -> (-8.7576, -25.479)
  line L116 (-8.7576, -25.479) -> (-8.7576, -25.8358)
  line L117 (-8.7576, -25.8358) -> (-8.971, -25.8358)
  spline S139 degree 2 poles (-8.971, -25.8358) (-8.7256, -26.0248) (-8.7256, -26.3129) knots 0 0 0 1 1 1
  spline S140 degree 2 poles (-8.7256, -26.3129) (-8.7256, -26.4409) (-8.8171, -26.6513) (-8.9588, -26.758) (-9.1387, -26.8007) (-9.3064, -26.8007) knots 0 0 0 1 2 3 4 4 4
  line L118 (-9.3064, -26.8007) -> (-10.2073, -26.8007)
  line L119 (-8.7576, -27.854) -> (-9.0625, -27.854)
  line L120 (-9.0625, -27.854) -> (-9.0625, -27.5919)
  line L121 (-9.0625, -27.5919) -> (-9.6463, -27.5919)
  spline S141 degree 2 poles (-9.6463, -27.5919) (-9.8231, -27.5919) (-9.8826, -27.6071) (-9.9207, -27.6604) (-9.9207, -27.6986) knots 0 0 0 1 2 3 3 3
  spline S142 degree 2 poles (-9.9207, -27.6986) (-9.9207, -27.7519) (-9.8841, -27.854) knots 0 0 0 1 1 1
  line L122 (-9.8841, -27.854) -> (-10.1814, -27.8861)
  spline S143 degree 2 poles (-10.1814, -27.8861) (-10.2393, -27.7519) (-10.2393, -27.5827) knots 0 0 0 1 1 1
  spline S144 degree 2 poles (-10.2393, -27.5827) (-10.2393, -27.479) (-10.1692, -27.3129) (-10.0594, -27.2351) (-9.9649, -27.2199) knots 0 0 0 1 2 3 3 3
  spline S145 degree 2 poles (-9.9649, -27.2199) (-9.8978, -27.2077) (-9.6951, -27.2077) knots 0 0 0 1 1 1
  line L123 (-9.6951, -27.2077) -> (-9.0625, -27.2077)
  line L124 (-9.0625, -27.2077) -> (-9.0625, -27.0324)
  line L125 (-9.0625, -27.0324) -> (-8.7576, -27.0324)
  line L126 (-8.7576, -27.0324) -> (-8.7576, -27.2077)
  line L127 (-8.7576, -27.2077) -> (-8.4695, -27.2077)
  line L128 (-8.4695, -27.2077) -> (-8.2439, -27.5919)
  line L129 (-8.2439, -27.5919) -> (-8.7576, -27.5919)
  line L130 (-8.7576, -27.5919) -> (-8.7576, -27.854)
  line L131 (-10.2073, -28.4882) -> (-10.2073, -28.104)
  line L132 (-10.2073, -28.104) -> (-8.7576, -28.104)
  line L133 (-8.7576, -28.104) -> (-8.7576, -28.4608)
  line L134 (-8.7576, -28.4608) -> (-8.9634, -28.4608)
  spline S146 degree 2 poles (-8.9634, -28.4608) (-8.8171, -28.5522) (-8.7256, -28.697) (-8.7256, -28.79) knots 0 0 0 1 2 2 2
  spline S147 degree 2 poles (-8.7256, -28.79) (-8.7256, -28.9211) (-8.7988, -29.0415) knots 0 0 0 1 1 1
  line L135 (-8.7988, -29.0415) -> (-9.1326, -28.9242)
  spline S148 degree 2 poles (-9.1326, -28.9242) (-9.0701, -28.8266) (-9.0701, -28.7443) knots 0 0 0 1 1 1
  spline S149 degree 2 poles (-9.0701, -28.7443) (-9.0701, -28.6635) (-9.1585, -28.5522) (-9.3902, -28.4882) (-9.7606, -28.4882) knots 0 0 0 1 2 3 3 3
  line L136 (-9.7606, -28.4882) -> (-10.2073, -28.4882)
  spline S150 degree 2 poles (-9.4619, -29.1178) (-9.2713, -29.1178) (-8.9131, -29.3068) (-8.7256, -29.6513) (-8.7256, -29.8647) knots 0 0 0 1 2 3 3 3
  spline S151 degree 2 poles (-8.7256, -29.8647) (-8.7256, -30.194) (-9.1524, -30.6147) (-9.4786, -30.6147) knots 0 0 0 1 2 2 2
  spline S152 degree 2 poles (-9.4786, -30.6147) (-9.8064, -30.6147) (-10.2393, -30.1894) (-10.2393, -29.8678) knots 0 0 0 1 2 2 2
  spline S153 degree 2 poles (-10.2393, -29.8678) (-10.2393, -29.6681) (-10.0594, -29.3068) (-9.7119, -29.1178) (-9.4619, -29.1178) knots 0 0 0 1 2 3 3 3
  spline S154 degree 2 poles (-9.4817, -29.5111) (-9.6981, -29.5111) (-9.9268, -29.7153) (-9.9268, -29.8662) knots 0 0 0 1 2 2 2
  spline S155 degree 2 poles (-9.9268, -29.8662) (-9.9268, -30.0172) (-9.6981, -30.2199) (-9.4802, -30.2199) knots 0 0 0 1 2 2 2
  spline S156 degree 2 poles (-9.4802, -30.2199) (-9.2667, -30.2199) (-9.0381, -30.0172) (-9.0381, -29.8662) knots 0 0 0 1 2 2 2
  spline S157 degree 2 poles (-9.0381, -29.8662) (-9.0381, -29.7153) (-9.2667, -29.5111) (-9.4817, -29.5111) knots 0 0 0 1 2 2 2
  line L137 (-10.2073, -30.915) -> (-8.2073, -30.915)
  line L138 (-8.2073, -30.915) -> (-8.2073, -31.2992)
  line L139 (-8.2073, -31.2992) -> (-10.2073, -31.2992)
  line L140 (-10.2073, -31.2992) -> (-10.2073, -30.915)
  line L141 (-9.9619, -34.2382) -> (-10.2591, -34.0065)
  spline S158 degree 2 poles (-10.2591, -34.0065) (-10.1753, -33.8358) (-10.0289, -33.6787) knots 0 0 0 1 1 1
  spline S159 degree 2 poles (-10.0289, -33.6787) (-10.1387, -33.5583) (-10.2424, -33.2854) (-10.2424, -33.0964) knots 0 0 0 1 2 2 2
  spline S160 degree 2 poles (-10.2424, -33.0964) (-10.2424, -32.7229) (-10.032, -32.5354) knots 0 0 0 1 1 1
  spline S161 degree 2 poles (-10.032, -32.5354) (-9.8704, -32.3891) (-9.6585, -32.3891) knots 0 0 0 1 1 1
  spline S162 degree 2 poles (-9.6585, -32.3891) (-9.4664, -32.3891) (-9.1585, -32.6178) (-9.0457, -32.8464) knots 0 0 0 1 2 2 2
  spline S163 degree 2 poles (-9.0457, -32.8464) (-8.9253, -32.7443) (-8.7058, -32.6406) (-8.6067, -32.6406) knots 0 0 0 1 2 2 2
  spline S164 degree 2 poles (-8.6067, -32.6406) (-8.4253, -32.6406) (-8.1738, -32.9318) (-8.1738, -33.2001) knots 0 0 0 1 2 2 2
  spline S165 degree 2 poles (-8.1738, -33.2001) (-8.1738, -33.4592) (-8.4375, -33.7504) (-8.628, -33.7504) knots 0 0 0 1 2 2 2
  spline S166 degree 2 poles (-8.628, -33.7504) (-8.75, -33.7504) (-8.9664, -33.6071) (-9.1036, -33.3891) knots 0 0 0 1 2 2 2
  line L142 (-9.1036, -33.3891) -> (-9.4725, -33.665)
  spline S167 degree 2 poles (-9.4725, -33.665) (-9.3856, -33.7138) (-9.2469, -33.7489) knots 0 0 0 1 1 1
  line L143 (-9.2469, -33.7489) -> (-9.3247, -34.0949)
  spline S168 degree 2 poles (-9.3247, -34.0949) (-9.5076, -34.0431) (-9.6783, -33.9669) (-9.7363, -33.9242) knots 0 0 0 1 2 2 2
  spline S169 degree 2 poles (-9.7363, -33.9242) (-9.7957, -33.9882) (-9.939, -34.1909) (-9.9619, -34.2382) knots 0 0 0 1 2 2 2
  spline S170 degree 2 poles (-9.2911, -33.0461) (-9.3582, -32.9135) (-9.5457, -32.7824) (-9.6448, -32.7824) knots 0 0 0 1 2 2 2
  spline S171 degree 2 poles (-9.6448, -32.7824) (-9.7683, -32.7824) (-9.9253, -32.944) (-9.9253, -33.0812) knots 0 0 0 1 2 2 2
  spline S172 degree 2 poles (-9.9253, -33.0812) (-9.9253, -33.1711) (-9.8536, -33.3373) (-9.7728, -33.4348) knots 0 0 0 1 2 2 2
  line L144 (-9.7728, -33.4348) -> (-9.2911, -33.0461)
  line L145 (-8.875, -33.1955) -> (-8.7972, -33.2992)
  spline S173 degree 2 poles (-8.7972, -33.2992) (-8.7073, -33.4135) (-8.6204, -33.4135) knots 0 0 0 1 1 1
  spline S174 degree 2 poles (-8.6204, -33.4135) (-8.5472, -33.4135) (-8.4436, -33.3037) (-8.4436, -33.2092) knots 0 0 0 1 2 2 2
  spline S175 degree 2 poles (-8.4436, -33.2092) (-8.4436, -33.1178) (-8.535, -33.0141) (-8.5945, -33.0141) knots 0 0 0 1 2 2 2
  spline S176 degree 2 poles (-8.5945, -33.0141) (-8.6661, -33.0141) (-8.7667, -33.101) knots 0 0 0 1 1 1
  line L146 (-8.7667, -33.101) -> (-8.875, -33.1955)
  spline S177 degree 2 poles (-9.2195, -35.1818) (-8.9146, -35.1818) (-8.7073, -35.2733) knots 0 0 0 1 1 1
  spline S178 degree 2 poles (-8.7073, -35.2733) (-8.5549, -35.3419) (-8.311, -35.5781) (-8.253, -35.7184) knots 0 0 0 1 2 2 2
  spline S179 degree 2 poles (-8.253, -35.7184) (-8.1738, -35.9044) (-8.1738, -36.1498) knots 0 0 0 1 1 1
  spline S180 degree 2 poles (-8.1738, -36.1498) (-8.1738, -36.5919) (-8.7225, -37.1223) (-9.2103, -37.1223) knots 0 0 0 1 2 2 2
  spline S181 degree 2 poles (-9.2103, -37.1223) (-9.6936, -37.1223) (-10.2408, -36.5949) (-10.2408, -36.1544) knots 0 0 0 1 2 2 2
  spline S182 degree 2 poles (-10.2408, -36.1544) (-10.2408, -35.7092) (-9.6966, -35.1818) (-9.2195, -35.1818) knots 0 0 0 1 2 2 2
  spline S183 degree 2 poles (-9.2058, -35.5979) (-9.5457, -35.5979) (-9.8963, -35.912) (-9.8963, -36.1544) knots 0 0 0 1 2 2 2
  spline S184 degree 2 poles (-9.8963, -36.1544) (-9.8963, -36.3967) (-9.5488, -36.7062) (-9.2012, -36.7062) knots 0 0 0 1 2 2 2
  spline S185 degree 2 poles (-9.2012, -36.7062) (-8.8567, -36.7062) (-8.5183, -36.4044) (-8.5183, -36.1544) knots 0 0 0 1 2 2 2
  spline S186 degree 2 poles (-8.5183, -36.1544) (-8.5183, -35.9044) (-8.8613, -35.5979) (-9.2058, -35.5979) knots 0 0 0 1 2 2 2
  line L147 (-8.7576, -38.0979) -> (-9.0625, -38.0979)
  line L148 (-9.0625, -38.0979) -> (-9.0625, -37.8358)
  line L149 (-9.0625, -37.8358) -> (-9.6463, -37.8358)
  spline S187 degree 2 poles (-9.6463, -37.8358) (-9.8231, -37.8358) (-9.8826, -37.851) (-9.9207, -37.9044) (-9.9207, -37.9425) knots 0 0 0 1 2 3 3 3
  spline S188 degree 2 poles (-9.9207, -37.9425) (-9.9207, -37.9958) (-9.8841, -38.0979) knots 0 0 0 1 1 1
  line L150 (-9.8841, -38.0979) -> (-10.1814, -38.13)
  spline S189 degree 2 poles (-10.1814, -38.13) (-10.2393, -37.9958) (-10.2393, -37.8266) knots 0 0 0 1 1 1
  spline S190 degree 2 poles (-10.2393, -37.8266) (-10.2393, -37.7229) (-10.1692, -37.5568) (-10.0594, -37.479) (-9.9649, -37.4638) knots 0 0 0 1 2 3 3 3
  spline S191 degree 2 poles (-9.9649, -37.4638) (-9.8978, -37.4516) (-9.6951, -37.4516) knots 0 0 0 1 1 1
  line L151 (-9.6951, -37.4516) -> (-9.0625, -37.4516)
  line L152 (-9.0625, -37.4516) -> (-9.0625, -37.2763)
  line L153 (-9.0625, -37.2763) -> (-8.7576, -37.2763)
  line L154 (-8.7576, -37.2763) -> (-8.7576, -37.4516)
  line L155 (-8.7576, -37.4516) -> (-8.4695, -37.4516)
  line L156 (-8.4695, -37.4516) -> (-8.2439, -37.8358)
  line L157 (-8.2439, -37.8358) -> (-8.7576, -37.8358)
  line L158 (-8.7576, -37.8358) -> (-8.7576, -38.0979)
  spline S192 degree 2 poles (-9.4619, -38.2748) (-9.2713, -38.2748) (-8.9131, -38.4638) (-8.7256, -38.8083) (-8.7256, -39.0217) knots 0 0 0 1 2 3 3 3
  spline S193 degree 2 poles (-8.7256, -39.0217) (-8.7256, -39.351) (-9.1524, -39.7717) (-9.4786, -39.7717) knots 0 0 0 1 2 2 2
  spline S194 degree 2 poles (-9.4786, -39.7717) (-9.8064, -39.7717) (-10.2393, -39.3464) (-10.2393, -39.0248) knots 0 0 0 1 2 2 2
  spline S195 degree 2 poles (-10.2393, -39.0248) (-10.2393, -38.8251) (-10.0594, -38.4638) (-9.7119, -38.2748) (-9.4619, -38.2748) knots 0 0 0 1 2 3 3 3
  spline S196 degree 2 poles (-9.4817, -38.6681) (-9.6981, -38.6681) (-9.9268, -38.8723) (-9.9268, -39.0233) knots 0 0 0 1 2 2 2
  spline S197 degree 2 poles (-9.9268, -39.0233) (-9.9268, -39.1742) (-9.6981, -39.3769) (-9.4802, -39.3769) knots 0 0 0 1 2 2 2
  spline S198 degree 2 poles (-9.4802, -39.3769) (-9.2667, -39.3769) (-9.0381, -39.1742) (-9.0381, -39.0233) knots 0 0 0 1 2 2 2
  spline S199 degree 2 poles (-9.0381, -39.0233) (-9.0381, -38.8723) (-9.2667, -38.6681) (-9.4817, -38.6681) knots 0 0 0 1 2 2 2
  line L159 (-8.7576, -40.0431) -> (-8.7576, -40.3967)
  line L160 (-8.7576, -40.3967) -> (-8.9558, -40.3967)
  spline S200 degree 2 poles (-8.9558, -40.3967) (-8.7256, -40.5873) (-8.7256, -40.8495) knots 0 0 0 1 1 1
  spline S201 degree 2 poles (-8.7256, -40.8495) (-8.7256, -40.9882) (-8.8399, -41.1925) (-8.9558, -41.258) knots 0 0 0 1 2 2 2
  spline S202 degree 2 poles (-8.9558, -41.258) (-8.8399, -41.354) (-8.7256, -41.5751) (-8.7256, -41.7001) knots 0 0 0 1 2 2 2
  spline S203 degree 2 poles (-8.7256, -41.7001) (-8.7256, -41.8601) (-8.8552, -42.0812) (-8.9802, -42.1361) knots 0 0 0 1 2 2 2
  spline S204 degree 2 poles (-8.9802, -42.1361) (-9.0731, -42.1757) (-9.2805, -42.1757) knots 0 0 0 1 1 1
  line L161 (-9.2805, -42.1757) -> (-10.2073, -42.1757)
  line L162 (-10.2073, -42.1757) -> (-10.2073, -41.7915)
  line L163 (-10.2073, -41.7915) -> (-9.378, -41.7915)
  spline S205 degree 2 poles (-9.378, -41.7915) (-9.1631, -41.7915) (-9.1006, -41.7519) knots 0 0 0 1 1 1
  spline S206 degree 2 poles (-9.1006, -41.7519) (-9.0183, -41.6986) (-9.0183, -41.5888) knots 0 0 0 1 1 1
  spline S207 degree 2 poles (-9.0183, -41.5888) (-9.0183, -41.508) (-9.1158, -41.3662) (-9.3064, -41.3037) (-9.5106, -41.3037) knots 0 0 0 1 2 3 3 3
  line L164 (-9.5106, -41.3037) -> (-10.2073, -41.3037)
  line L165 (-10.2073, -41.3037) -> (-10.2073, -40.9196)
  line L166 (-10.2073, -40.9196) -> (-9.4131, -40.9196)
  spline S208 degree 2 poles (-9.4131, -40.9196) (-9.2012, -40.9196) (-9.0777, -40.8784) (-9.0183, -40.7931) (-9.0183, -40.7184) knots 0 0 0 1 2 3 3 3
  spline S209 degree 2 poles (-9.0183, -40.7184) (-9.0183, -40.63) (-9.1143, -40.4882) (-9.2942, -40.4272) (-9.503, -40.4272) knots 0 0 0 1 2 3 3 3
  line L167 (-9.503, -40.4272) -> (-10.2073, -40.4272)
  line L168 (-10.2073, -40.4272) -> (-10.2073, -40.0431)
  line L169 (-10.2073, -40.0431) -> (-8.7576, -40.0431)
  line L170 (-9.1997, -42.8419) -> (-9.1372, -42.4943)
  spline S210 degree 2 poles (-9.1372, -42.4943) (-8.9268, -42.5537) (-8.7256, -42.8403) (-8.7256, -43.1223) knots 0 0 0 1 2 2 2
  spline S211 degree 2 poles (-8.7256, -43.1223) (-8.7256, -43.38) (-8.8475, -43.6315) (-9.0335, -43.7336) (-9.2835, -43.7336) knots 0 0 0 1 2 3 3 3
  line L171 (-9.2835, -43.7336) -> (-9.7317, -43.7275)
  spline S212 degree 2 poles (-9.7317, -43.7275) (-9.9222, -43.7275) (-10.1036, -43.7641) (-10.2073, -43.8144) knots 0 0 0 1 2 2 2
  line L172 (-10.2073, -43.8144) -> (-10.2073, -43.4348)
  spline S213 degree 2 poles (-10.2073, -43.4348) (-10.1692, -43.4196) (-10.0945, -43.3983) knots 0 0 0 1 1 1
  spline S214 degree 2 poles (-10.0945, -43.3983) (-10.0594, -43.3891) (-10.0488, -43.3845) knots 0 0 0 1 1 1
  spline S215 degree 2 poles (-10.0488, -43.3845) (-10.1433, -43.287) (-10.2393, -43.0629) (-10.2393, -42.9364) knots 0 0 0 1 2 2 2
  spline S216 degree 2 poles (-10.2393, -42.9364) (-10.2393, -42.7123) (-9.9969, -42.4547) (-9.811, -42.4547) knots 0 0 0 1 2 2 2
  spline S217 degree 2 poles (-9.811, -42.4547) (-9.6875, -42.4547) (-9.4954, -42.572) (-9.3933, -42.7839) (-9.3552, -42.9836) knots 0 0 0 1 2 3 3 3
  spline S218 degree 2 poles (-9.3552, -42.9836) (-9.3049, -43.2519) (-9.2606, -43.3556) knots 0 0 0 1 1 1
  line L173 (-9.2606, -43.3556) -> (-9.2225, -43.3556)
  spline S219 degree 2 poles (-9.2225, -43.3556) (-9.1128, -43.3556) (-9.0183, -43.2458) (-9.0183, -43.0949) knots 0 0 0 1 2 2 2
  spline S220 degree 2 poles (-9.0183, -43.0949) (-9.0183, -42.9928) (-9.0991, -42.8769) (-9.1997, -42.8419) knots 0 0 0 1 2 2 2
  spline S221 degree 2 poles (-9.5106, -43.3556) (-9.535, -43.2824) (-9.6036, -42.9623) (-9.6356, -42.9135) knots 0 0 0 1 2 2 2
  spline S222 degree 2 poles (-9.6356, -42.9135) (-9.689, -42.8388) (-9.7713, -42.8388) knots 0 0 0 1 1 1
  spline S223 degree 2 poles (-9.7713, -42.8388) (-9.8521, -42.8388) (-9.9695, -42.9592) (-9.9695, -43.0522) knots 0 0 0 1 2 2 2
  spline S224 degree 2 poles (-9.9695, -43.0522) (-9.9695, -43.1559) (-9.9009, -43.2489) knots 0 0 0 1 1 1
  spline S225 degree 2 poles (-9.9009, -43.2489) (-9.8491, -43.319) (-9.7744, -43.3403) knots 0 0 0 1 1 1
  spline S226 degree 2 poles (-9.7744, -43.3403) (-9.7256, -43.3556) (-9.5869, -43.3556) knots 0 0 0 1 1 1
  line L174 (-9.5869, -43.3556) -> (-9.5106, -43.3556)
  line L175 (-9.7927, -43.9745) -> (-9.7347, -44.3586)
  spline S227 degree 2 poles (-9.7347, -44.3586) (-9.846, -44.383) (-9.9619, -44.5339) (-9.9619, -44.6681) knots 0 0 0 1 2 2 2
  spline S228 degree 2 poles (-9.9619, -44.6681) (-9.9619, -44.8175) (-9.907, -44.8922) knots 0 0 0 1 1 1
  spline S229 degree 2 poles (-9.907, -44.8922) (-9.8689, -44.9425) (-9.8049, -44.9425) knots 0 0 0 1 1 1
  spline S230 degree 2 poles (-9.8049, -44.9425) (-9.7622, -44.9425) (-9.7332, -44.915) knots 0 0 0 1 1 1
  spline S231 degree 2 poles (-9.7332, -44.915) (-9.7058, -44.8861) (-9.6829, -44.787) knots 0 0 0 1 1 1
  spline S232 degree 2 poles (-9.6829, -44.787) (-9.5808, -44.3236) (-9.4954, -44.2001) knots 0 0 0 1 1 1
  spline S233 degree 2 poles (-9.4954, -44.2001) (-9.378, -44.0278) (-9.1707, -44.0278) knots 0 0 0 1 1 1
  spline S234 degree 2 poles (-9.1707, -44.0278) (-8.9817, -44.0278) (-8.7256, -44.3251) (-8.7256, -44.6376) knots 0 0 0 1 2 2 2
  spline S235 degree 2 poles (-8.7256, -44.6376) (-8.7256, -44.9348) (-8.9192, -45.2229) (-9.1097, -45.2778) knots 0 0 0 1 2 2 2
  line L176 (-9.1097, -45.2778) -> (-9.1768, -44.9165)
  spline S236 degree 2 poles (-9.1768, -44.9165) (-9.0914, -44.8937) (-9.0015, -44.7641) (-9.0015, -44.6437) knots 0 0 0 1 2 2 2
  spline S237 degree 2 poles (-9.0015, -44.6437) (-9.0015, -44.4928) (-9.0442, -44.4287) knots 0 0 0 1 1 1
  spline S238 degree 2 poles (-9.0442, -44.4287) (-9.0731, -44.3845) (-9.1219, -44.3845) knots 0 0 0 1 1 1
  spline S239 degree 2 poles (-9.1219, -44.3845) (-9.1616, -44.3845) (-9.1905, -44.4226) knots 0 0 0 1 1 1
  spline S240 degree 2 poles (-9.1905, -44.4226) (-9.2286, -44.4745) (-9.3674, -45.0858) (-9.4695, -45.2062) knots 0 0 0 1 2 2 2
  spline S241 degree 2 poles (-9.4695, -45.2062) (-9.5716, -45.3266) (-9.7546, -45.3266) knots 0 0 0 1 1 1
  spline S242 degree 2 poles (-9.7546, -45.3266) (-9.9527, -45.3266) (-10.2393, -44.9943) (-10.2393, -44.6681) knots 0 0 0 1 2 2 2
  spline S243 degree 2 poles (-10.2393, -44.6681) (-10.2393, -44.3723) (-9.9985, -44.0278) (-9.7927, -43.9745) knots 0 0 0 1 2 2 2
  line L177 (-10.2073, -45.6635) -> (-8.7576, -45.6635)
  line L178 (-8.7576, -45.6635) -> (-8.7576, -46.0476)
  line L179 (-8.7576, -46.0476) -> (-10.2073, -46.0476)
  line L180 (-10.2073, -46.0476) -> (-10.2073, -45.6635)
  line L181 (-8.5625, -45.6635) -> (-8.2073, -45.6635)
  line L182 (-8.2073, -45.6635) -> (-8.2073, -46.0476)
  line L183 (-8.2073, -46.0476) -> (-8.5625, -46.0476)
  line L184 (-8.5625, -46.0476) -> (-8.5625, -45.6635)
  line L185 (-12.998, -28.944) -> (-13.3547, -28.944)
  line L186 (-13.3547, -28.944) -> (-13.3547, -27.601)
  spline S244 degree 2 poles (-13.3547, -27.601) (-13.1535, -27.6223) (-12.7922, -27.8403) (-12.4934, -28.1635) knots 0 0 0 1 2 2 2
  spline S245 degree 2 poles (-12.4934, -28.1635) (-12.2526, -28.4226) (-12.1657, -28.4806) knots 0 0 0 1 1 1
  spline S246 degree 2 poles (-12.1657, -28.4806) (-12.0468, -28.5598) (-11.9309, -28.5598) knots 0 0 0 1 1 1
  spline S247 degree 2 poles (-11.9309, -28.5598) (-11.8029, -28.5598) (-11.6657, -28.4226) (-11.6657, -28.3007) knots 0 0 0 1 2 2 2
  spline S248 degree 2 poles (-11.6657, -28.3007) (-11.6657, -28.1818) (-11.8105, -28.04) (-11.9782, -28.0294) knots 0 0 0 1 2 2 2
  line L187 (-11.9782, -28.0294) -> (-11.9401, -27.6467)
  spline S249 degree 2 poles (-11.9401, -27.6467) (-11.623, -27.6803) (-11.3471, -28.04) (-11.3471, -28.3098) knots 0 0 0 1 2 2 2
  spline S250 degree 2 poles (-11.3471, -28.3098) (-11.3471, -28.6056) (-11.6657, -28.944) (-11.9035, -28.944) knots 0 0 0 1 2 2 2
  spline S251 degree 2 poles (-11.9035, -28.944) (-12.0376, -28.944) (-12.2815, -28.8479) (-12.4157, -28.7428) knots 0 0 0 1 2 2 2
  spline S252 degree 2 poles (-12.4157, -28.7428) (-12.5041, -28.6726) (-12.8364, -28.3098) (-12.9462, -28.2123) (-12.998, -28.1833) knots 0 0 0 1 2 3 3 3
  line L188 (-12.998, -28.1833) -> (-12.998, -28.944)
  spline S253 degree 2 poles (-11.3471, -29.851) (-11.3471, -30.1422) (-11.5544, -30.3053) knots 0 0 0 1 1 1
  spline S254 degree 2 poles (-11.5544, -30.3053) (-11.7998, -30.5004) (-12.3684, -30.5004) knots 0 0 0 1 1 1
  spline S255 degree 2 poles (-12.3684, -30.5004) (-12.9355, -30.5004) (-13.184, -30.3037) knots 0 0 0 1 1 1
  spline S256 degree 2 poles (-13.184, -30.3037) (-13.3882, -30.1422) (-13.3882, -29.851) knots 0 0 0 1 1 1
  spline S257 degree 2 poles (-13.3882, -29.851) (-13.3882, -29.5583) (-12.9401, -29.2016) (-12.3638, -29.2016) knots 0 0 0 1 2 2 2
  spline S258 degree 2 poles (-12.3638, -29.2016) (-11.7998, -29.2016) (-11.5513, -29.3983) knots 0 0 0 1 1 1
  spline S259 degree 2 poles (-11.5513, -29.3983) (-11.3471, -29.5598) (-11.3471, -29.851) knots 0 0 0 1 1 1